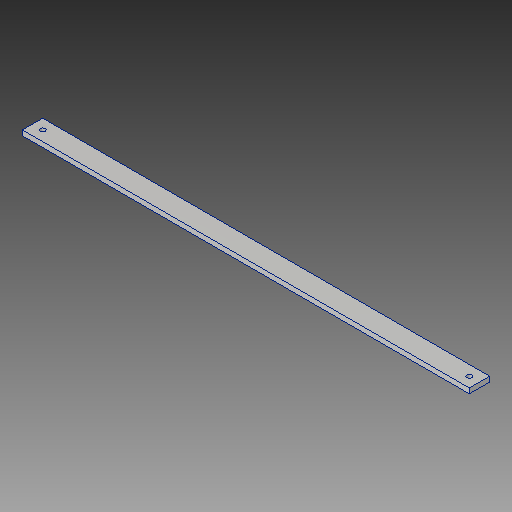
# Autodesk Inventor part: 15102898-16-P-0214
Saved by Autodesk Inventor 2017 (Build 210142000, 142)
## iProperties
Created: 2016-10-05
Part Number: 15102898-16-P-0214
Material: Aluminum 6061
Document SubType Name: Sheet Metal
Designer: gus
Density: 2.7 g/cm^3
Appearance: Aluminum - Flat
Sheet Metal Rule: Default
Mass: 242.262 g
Surface Area: 359.331 cm^2
Volume: 89.7267 cm^3
Author: gus
Autodesk Inventor part; units mm, degrees
ref_plane "YZ Plane" through (0, 0, 0) normal (1, 0, 0) x (0, 1, 0)
ref_plane "XZ Plane" through (0, 0, 0) normal (0, 1, 0) x (-1, 0, 0)
ref_plane "XY Plane" through (0, 0, 0) normal (0, 0, 1) x (1, 0, 0)
sketch "Sketch1" plane through (0, 0, 0) normal (0, 1, 0) x (-1, 0, 0)
  line L0 (0, 0) -> (-558.8, 0)
  line L1 (-558.8, 0) -> (-558.8, 25.4)
  line L2 (-558.8, 25.4) -> (0, 25.4)
  line L3 (0, 25.4) -> (0, 0)
  circle A0 centre (-12.7, 12.7) radius 3.175
  circle A1 centre (-546.1, 12.7) radius 3.175
  dimension "d0" = 558.8
  dimension "d1" = 25.4
  dimension "d2" = 6.35
  dimension "d3" = 12.7
  dimension "d4" = 12.7
  dimension "d5" = 6.35
  dimension "d6" = 12.7
  dimension "d7" = 12.7
  constraints: 8 end point, 2 centre point, 2 parallel, 1 horizontal, 1 perpendicular
  measures "d0" distance of L1.end L2.end
  measures "d1" distance of L0.end L1.end
  measures "d2" diameter of A0
  measures "d3" distance from line of L0 A0.centre
  measures "d4" distance from line of L3 A0.centre
  measures "d5" diameter of A1
  measures "d6" distance from line of L1 A1.centre
  measures "d7" distance from line of L0 A1.centre
extrude "Extrusion1" add sketch "Sketch1" along normal blind 6.35
equation "\"BendRadius\" = Thickness"
equation "\"BendReliefWidth\" = Thickness"
equation "\"BendReliefDepth\" = 0.5 * Thickness"
equation "\"CornerReliefSize\" = 4 * Thickness"
equation "\"MinimumRemnant\" = 2 * Thickness"
equation "\"TransitionRadius\" = BendRadius"
equation "\"JacobiRadiusSize\" = Thickness"
equation "\"GapSize\" = Thickness"
equation "\"Thickness\" = 3.048"
body "Solid1"
